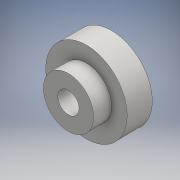
# Autodesk Inventor part: HeadBarClampTurnwheel
Saved by Autodesk Inventor 2016 (Build 200138000, 138)
## iProperties
Created: 2015-11-18
Part Number: HeadBarClampTurnwheel
Material: UHMW, White
Document SubType Name: Modeling
Designer: Vervaeke-Lab
Mass: 0.871458 g
Surface Area: 7.32337 cm^2
Volume: 0.927083 cm^3
Density: 0.94 g/cm^3
Appearance: Smooth - White
Author: Vervaeke-Lab
Autodesk Inventor part; units mm, degrees
ref_plane "YZ Plane" through (0, 0, 0) normal (1, 0, 0) x (0, 1, 0)
ref_plane "XZ Plane" through (0, 0, 0) normal (0, 1, 0) x (-1, 0, 0)
ref_plane "XY Plane" through (0, 0, 0) normal (0, 0, 1) x (1, 0, 0)
sketch "Sketch1" plane through (0, 0, 0) normal (0, 1, 0) x (-1, 0, 0)
  circle A0 centre (0, 0) radius 7.45
  dimension "d0" = 14.9
  constraints: 1 centre point, 1 coincident
  measures "d0" diameter of A0
extrude "Extrusion1" add sketch "Sketch1" along normal blind 7.9
sketch "Sketch2" plane through (0, 0, 0) normal (0, 1, 0) x (-1, 0, 0)
  circle A0 centre (0, 0) radius 4.6
  circle A1 centre (0, 0) radius 7.45
  dimension "d3" = 9.2
  constraints: 2 centre point, 2 coincident
  measures "d3" diameter of A0
extrude "Extrusion2" cut sketch "Sketch2" along normal blind 3.3
sketch "Sketch3" plane through (0, 7.9, 0) normal (0, 1, 0) x (1, 0, 0)
  point P0 (0, 0)
  point P1 (0, 0)
  constraints: 1 coincident
hole "Hole1" at (0, 7.9, 0) direction (0, -1, 0) diameter 3.9 end through all
body "Solid1"
